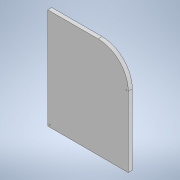
# Autodesk Inventor part: Dół
Saved by Autodesk Inventor 2022 (Build 260153000, 153)
## iProperties
Created: 2024-01-26
Part Number: Dół
Material: Generic
Document SubType Name: Modeling
Designer: mateu
Density: 1 g/cm^3
Appearance: Default
Author: mateu
Autodesk Inventor part; units mm, degrees
ref_plane "YZ Plane" through (0, 0, 0) normal (1, 0, 0) x (0, 1, 0)
ref_plane "XZ Plane" through (0, 0, 0) normal (0, 1, 0) x (-1, 0, 0)
ref_plane "XY Plane" through (0, 0, 0) normal (0, 0, 1) x (1, 0, 0)
sketch "Sketch1" plane through (0, 0, 0) normal (0, 0, 1) x (1, 0, 0)
  point P0 (0, 0)
sketch "Sketch2" plane through (0, 0, 0) normal (0, 0, 1) x (1, 0, 0)
  line L0 (0, 0) -> (40, 0)
  line L1 (40, 0) -> (40, 50)
  line L2 (40, 50) -> (0, 50)
  line L3 (0, 50) -> (0, 0)
  constraints: 8 end point, 3 perpendicular, 1 horizontal
extrude "Extrusion1" add sketch "Sketch2" along normal blind 2
sketch "Sketch3" plane through (0, 0, 2) normal (0, 0, 1) x (1, 0, 0)
  point P0 (0, 0)
fillet "Fillet1" radius 15 1 edges at (40, 50, 1)
sketch "Sketch4" plane through (0, 0, 2) normal (0, 0, 1) x (1, 0, 0)
  point P0 (0, 0)
  point P1 (1, 1)
  point P2 (39, 35)
hole "Hole1" at (1, 1, 2) direction (0, 0, -1) diameter 0.37 end through all thread size "M0.5x0.125" class "6H" standard "ISO Metric profile"
sketch "Sketch5" plane through (0, 0, 2) normal (0, 0, 1) x (1, 0, 0)
  point P0 (0, 0)
  point P1 (39, 35)
hole "Hole2" at (39, 35, 2) direction (0, 0, -1) diameter 0.37 end through all thread size "M0.5x0.125" class "6H" standard "ISO Metric profile"
body "Solid1"
